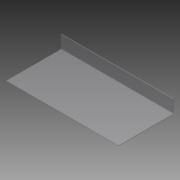
# Autodesk Inventor part: battery holder poly
Saved by Autodesk Inventor 2014 SP1 (Build 180222100, 222)
## iProperties
Created: 2014-04-06
Part Number: battery holder poly
Material: Generic
Document SubType Name: Modeling
Designer: Ryan
Density: 1 g/cm^3
Appearance: Polycarbonate - Clear
Author: Ryan
Autodesk Inventor part; units mm, degrees
note: some values were not read from the file. Chosen so that the rebuilt part matches the saved one: bend side of "Bend Part1".
ref_plane "YZ Plane" through (0, 0, 0) normal (1, 0, 0) x (0, 1, 0)
ref_plane "XZ Plane" through (0, 0, 0) normal (0, 1, 0) x (-1, 0, 0)
ref_plane "XY Plane" through (0, 0, 0) normal (0, 0, 1) x (1, 0, 0)
sketch "Sketch1" plane through (0, 0, 0) normal (0, 1, 0) x (-1, 0, 0)
  line L0 (-12.7612, -185.5673) -> (304.7388, -185.5673)
  line L1 (304.7388, -185.5673) -> (304.7388, 4.9327)
  line L2 (304.7388, 4.9327) -> (-12.7612, 4.9327)
  line L3 (-12.7612, 4.9327) -> (-12.7612, -185.5673)
  point P0 (0, 0)
  dimension "d0" = 317.5
  dimension "d1" = 190.5
  constraints: 8 end point, 2 parallel, 1 horizontal, 1 perpendicular
  measures "d0" distance of L2.end L1.end
  measures "d1" distance of L0.end L1.end
extrude "Extrusion1" add sketch "Sketch1" along normal blind 1.5875
sketch "Sketch2" plane through (0, 1.5875, 0) normal (0, 1, 0) x (1, 0, 0)
  line L0 (12.7612, 185.5673) -> (-304.7388, 185.5673) projected
  line L1 (12.7612, -4.9327) -> (12.7612, 185.5673) projected
  line L2 (-341.3221, 147.4673) -> (43.4131, 147.4673)
  point P0 (0, 0)
  dimension "d4" = 38.1
  constraints: 2 end point, 1 perpendicular
  measures "d4" distance between parallel lines of L0 L2
bend part "Bend Part1" radius 2.54 angle 90 line through (-341.3221, 1.5875, -147.4673) along (1, 0, 0) centre toward (0, 1, 0) moving side (0, 0, -1) both sides no
body "Solid1"
